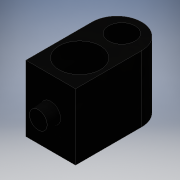
# Autodesk Inventor part: mocowanieDiod
Saved by Autodesk Inventor 2016 (Build 200138000, 138)
## iProperties
Created: 2017-06-11
Part Number: mocowanieDiod
Material: Ogólny
Document SubType Name: Modeling
Designer: Karol
Density: 1 g/cm^3
Appearance: Fine Textured - Black
Author: Karol
Autodesk Inventor part; units mm, degrees
ref_plane "YZ Plane" through (0, 0, 0) normal (1, 0, 0) x (0, 1, 0)
ref_plane "XZ Plane" through (0, 0, 0) normal (0, 1, 0) x (-1, 0, 0)
ref_plane "XY Plane" through (0, 0, 0) normal (0, 0, 1) x (1, 0, 0)
sketch "Szkic3" plane through (0, 0, 0) normal (0, 1, 0) x (-1, 0, 0)
  line L0 (3, 4) -> (-3, 4)
  line L1 (-3, 4) -> (-3, -4)
  line L2 (-3, -4) -> (3, -4)
  line L3 (3, -4) -> (3, 4)
  line L4 (3, 4) -> (-3, -4) construction
  line L5 (-3, 4) -> (3, -4) construction
  point P0 (0, 0)
  dimension "d8" = 6
  dimension "d9" = 8
  constraints: 12 end point, 2 midpoint, 2 parallel, 1 horizontal, 1 perpendicular
  measures "d8" distance of L1.end L2.end
  measures "d9" distance of L2.end L0.start
extrude "Wyciągnięcie proste2" add sketch "Szkic3" along normal blind 11
sketch "Szkic4" plane through (-3, 0, 4) normal (0, 0, 1) x (1, 0, 0)
  circle A0 centre (3, 3.5) radius 2.5
  line L0 (6, 0) -> (6, 11) projected
  line L1 (0, 0) -> (0, 11) projected
  circle A1 centre (3, 8.6) radius 1.6
  point P0 (3, 0)
  dimension "d12" = 5
  dimension "d13" = 3
  dimension "d14" = 3
  dimension "d15" = 3.5
  dimension "d16" = 3.2
  dimension "d17" = 5.1
  constraints: 2 centre point, 1 vertical alignment
  measures "d12" diameter of A0
  measures "d13" distance from line of A0.centre L0
  measures "d14" distance from line of L1 A0.centre
  measures "d15" distance of point (3, 0) A0.centre
  measures "d16" diameter of A1
  measures "d17" distance of A1.centre A0.centre
extrude "Wyciągnięcie proste3" cut sketch "Szkic4" against normal up to next contours A1
extrude "Wyciągnięcie proste4" cut sketch "Szkic4" against normal up to next draft -5 contours A0
sketch "Szkic5" plane through (0, 0, 0) normal (0, -1, 0) x (1, 0, 0)
  circle A0 centre (0, 0) radius 1.2
  dimension "d22" = 2.4
  constraints: 1 centre point, 1 coincident
  measures "d22" diameter of A0
extrude "Wyciągnięcie proste5" add sketch "Szkic5" along normal blind 1.5 draft -5
fillet "Fillet2" radius 3 2 edges at (-3, 11, 0) (3, 11, 0)
equation "\"d14\" = d13"
